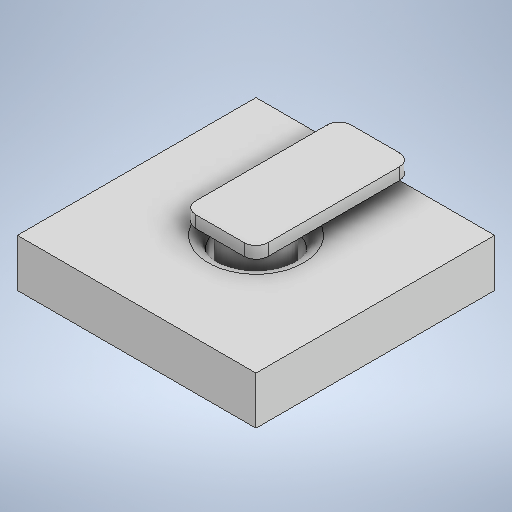
# Autodesk Inventor part: Lock
Saved by Autodesk Inventor 2025.2 (Build 292293000, 293)
## iProperties
Created: 2024-12-09
Part Number: Lock
Material: Generic
Document SubType Name: Modeling
Designer: jurre
Density: 1 g/cm^3
Appearance: Default
Author: jurre
Autodesk Inventor part; units mm, degrees
ref_plane "YZ Plane" through (0, 0, 0) normal (1, 0, 0) x (0, 1, 0)
ref_plane "XZ Plane" through (0, 0, 0) normal (0, 1, 0) x (-1, 0, 0)
ref_plane "XY Plane" through (0, 0, 0) normal (0, 0, 1) x (1, 0, 0)
sketch "Sketch1" plane through (0, 0, 0) normal (0, 1, 0) x (-1, 0, 0)
  line L0 (6.7863, 1.219) -> (-3.2137, 1.219)
  line L1 (-3.2137, 1.219) -> (-3.2137, -8.781)
  line L2 (-3.2137, -8.781) -> (6.7863, -8.781)
  line L3 (6.7863, -8.781) -> (6.7863, 1.219)
  circle A0 centre (1.7863, -3.781) radius 1.5
  point P0 (0, 0)
  dimension "d0" = 10
  dimension "d1" = 10
  dimension "d2" = 3
  constraints: 8 end point, 2 parallel, 1 centre point, 1 horizontal, 1 perpendicular
  measures "d0" distance of L2.end L1.end
  measures "d1" distance of L0.end L1.end
  measures "d2" diameter of A0
extrude "Extrusion1" add sketch "Sketch1" along normal blind 2
fillet "Fillet1" radius 0.5 1 edges at (-0.2863, 2, -3.781)
fillet "Fillet2" radius 0.5 1 edges at (-0.2863, 0, -3.781)
sketch "Sketch3" plane through (0, 0, 0) normal (0, 1, 0) x (-1, 0, 0)
  circle A0 centre (1.7863, -3.778) radius 1.25
  circle A1 centre (1.7863, -3.778) radius 1.75
  circle A2 centre (1.7863, -3.781) radius 1.5 projected
  point P0 (0, 0)
  dimension "d10" = 0
  dimension "d11" = 2.5
  dimension "d12" = 3.5
  constraints: 2 centre point, 1 coincident
  measures "d10" horizontal distance of A2.centre A0.centre
  measures "d11" diameter of A0
  measures "d12" diameter of A1
extrude "Extrusion2" add sketch "Sketch3" against normal blind 0.5 contours A0 | A1 | A2
extrude "Extrusion3" add sketch "Sketch3" along normal blind 2.5 contours A0
sketch "Sketch4" plane through (-1.7863, 2.5, -3.778) normal (0, 1, 0) x (1, 0, 0)
  line L0 (5, 5.003) -> (-5, 5.003) projected
  line L1 (-1.5134, -1.5105) -> (1.518, -1.5105)
  line L2 (1.518, -1.5105) -> (1.518, 5.003)
  line L3 (1.518, 5.003) -> (-1.5134, 5.003)
  line L4 (-1.5134, 5.003) -> (-1.5134, -1.5105)
  point P0 (1.7863, -3.778)
  constraints: 8 end point, 2 parallel, 1 horizontal, 1 perpendicular, 1 point on line
extrude "Extrusion4" add sketch "Sketch4" along normal blind 0.5
fillet "Fillet3" radius 0.5 4 edges at (-0.2683, 2.75, -2.2675) (-0.2683, 2.75, -8.781) (-3.2997, 2.75, -8.781) (-3.2997, 2.75, -2.2675)
fillet "Fillet4" radius 0.25 1 edges at (-0.0363, 0, -3.778)
sketch "Sketch5" plane through (-1.7863, -0.5, -3.778) normal (0, -1, 0) x (1, 0, 0)
  line L0 (-0.2331, -1.784) -> (0.2285, -1.784)
  line L1 (0.2285, -1.784) -> (0.2285, 1.842)
  line L2 (0.2285, 1.842) -> (-0.2331, 1.842)
  line L3 (-0.2331, 1.842) -> (-0.2331, -1.784)
  point P0 (1.7863, 3.778)
  constraints: 8 end point, 2 parallel, 1 horizontal, 1 perpendicular
extrude "Extrusion5" cut sketch "Sketch5" against normal blind 0.25
body "Solid1"
